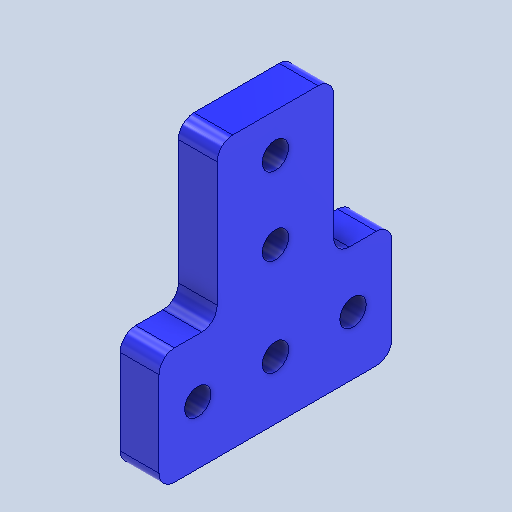
# Autodesk Inventor part: ball_loading_v1_Plate_ASP_F_1
Saved by Autodesk Inventor 2025.1 (Build 291241000, 241)
## iProperties
Created: 2024-11-12
Part Number: ball_loading_v1_Plate_ASP_F_1
Material: ABS プラスチック
Document SubType Name: Modeling
Designer: haruy
Density: 1.06 g/cm^3
Appearance: 青 - 壁塗料 - 光沢
Author: haruy
Autodesk Inventor part; units mm, degrees
ref_plane "YZ Plane" through (0, 0, 0) normal (1, 0, 0) x (0, 1, 0)
ref_plane "XZ Plane" through (0, 0, 0) normal (0, 1, 0) x (-1, 0, 0)
ref_plane "XY Plane" through (0, 0, 0) normal (0, 0, 1) x (1, 0, 0)
sketch "スケッチ1" plane through (0, 0, 0) normal (1, 0, 0) x (0, 1, 0)
  line L0 (-167.5617, 195.4399) -> (192.4383, 195.4399)
  line L1 (192.4383, 195.4399) -> (192.4383, 180.4399)
  line L2 (192.4383, 180.4399) -> (-167.5617, 180.4399)
  line L3 (-167.5617, 180.4399) -> (-167.5617, 195.4399)
  line L4 (-167.5617, 230.4399) -> (-182.5617, 230.4399)
  line L5 (-182.5617, 230.4399) -> (-182.5617, 2.9399)
  line L6 (-182.5617, 2.9399) -> (-167.5617, 2.9399)
  line L7 (-167.5617, 2.9399) -> (-167.5617, 230.4399)
  line L8 (-167.5617, 230.4399) -> (-182.5617, 230.4399)
  line L9 (-182.5617, 230.4399) -> (-182.5617, 215.4399)
  line L10 (-182.5617, 215.4399) -> (-167.5617, 215.4399)
  line L11 (-167.5617, 215.4399) -> (-167.5617, 230.4399)
  line L12 (-117.5617, 180.4399) -> (-102.5617, 180.4399)
  line L13 (-102.5617, 180.4399) -> (-102.5617, 2.9399)
  line L14 (-102.5617, 2.9399) -> (-117.5617, 2.9399)
  line L15 (-117.5617, 2.9399) -> (-117.5617, 180.4399)
  line L16 (192.4383, 180.4399) -> (177.4383, 180.4399)
  line L17 (177.4383, 180.4399) -> (177.4383, 2.9399)
  line L18 (177.4383, 2.9399) -> (192.4383, 2.9399)
  line L19 (192.4383, 2.9399) -> (192.4383, 180.4399)
  circle A0 centre (-142.5617, 135.4399) radius 12.5
  circle A1 centre (-142.5617, 95.4399) radius 18.75
  line L20 (192.4383, 2.9399) -> (-167.5617, 2.9399)
  line L21 (-182.5617, 155.4399) -> (-102.5617, 155.4399)
  line L22 (-102.5617, 75.4399) -> (-182.5617, 75.4399)
  circle A2 centre (-142.5617, 95.4399) radius 20
  line L23 (-125.0617, 195.4399) -> (-125.0617, 180.4399)
  line L24 (-102.5617, 180.4399) -> (-102.5617, 195.4399)
  line L25 (-147.5617, 195.4399) -> (-147.5617, 180.4399)
  line L26 (-167.5617, 202.9399) -> (-182.5617, 202.9399)
  line L27 (-167.5617, 172.9399) -> (-182.5617, 172.9399)
  circle A3 centre (157.4383, 135.4399) radius 12.5
  line L28 (192.4383, 160.4399) -> (177.4383, 160.4399)
  line L29 (169.9383, 195.4399) -> (169.9383, 180.4399)
  line L30 (-167.5617, -189.5601) -> (192.4383, -189.5601)
  line L31 (192.4383, -189.5601) -> (192.4383, -174.5601)
  line L32 (192.4383, -174.5601) -> (-167.5617, -174.5601)
  line L33 (-167.5617, -174.5601) -> (-167.5617, -189.5601)
  line L34 (-167.5617, -224.5601) -> (-182.5617, -224.5601)
  line L35 (-182.5617, -224.5601) -> (-182.5617, 2.9399)
  line L36 (-167.5617, 2.9399) -> (-167.5617, -224.5601)
  line L37 (-167.5617, -224.5601) -> (-182.5617, -224.5601)
  line L38 (-182.5617, -224.5601) -> (-182.5617, -209.5601)
  line L39 (-182.5617, -209.5601) -> (-167.5617, -209.5601)
  line L40 (-167.5617, -209.5601) -> (-167.5617, -224.5601)
  line L41 (-117.5617, -174.5601) -> (-102.5617, -174.5601)
  line L42 (-102.5617, -174.5601) -> (-102.5617, 2.9399)
  line L43 (-117.5617, 2.9399) -> (-117.5617, -174.5601)
  line L44 (192.4383, -174.5601) -> (177.4383, -174.5601)
  line L45 (177.4383, -174.5601) -> (177.4383, 2.9399)
  line L46 (192.4383, 2.9399) -> (192.4383, -174.5601)
  circle A4 centre (-142.5617, -129.5601) radius 12.5
  circle A5 centre (-142.5617, -89.5601) radius 18.75
  line L47 (-182.5617, -149.5601) -> (-102.5617, -149.5601)
  line L48 (-102.5617, -69.5601) -> (-182.5617, -69.5601)
  circle A6 centre (-142.5617, -89.5601) radius 20
  line L49 (-125.0617, -189.5601) -> (-125.0617, -174.5601)
  line L50 (-102.5617, -174.5601) -> (-102.5617, -189.5601)
  line L51 (-147.5617, -189.5601) -> (-147.5617, -174.5601)
  line L52 (-167.5617, -197.0601) -> (-182.5617, -197.0601)
  line L53 (-167.5617, -167.0601) -> (-182.5617, -167.0601)
  circle A7 centre (157.4383, -129.5601) radius 12.5
  line L54 (192.4383, -154.5601) -> (177.4383, -154.5601)
  line L55 (169.9383, -189.5601) -> (169.9383, -174.5601)
  line L56 (192.4383, 155.4399) -> (144.9383, 155.4399)
  line L57 (144.9383, 155.4399) -> (144.9383, 75.4399)
  line L58 (144.9383, 75.4399) -> (192.4383, 75.4399)
  line L59 (192.4383, 75.4399) -> (192.4383, 155.4399)
  line L60 (177.4383, 155.4399) -> (153.4158, 147.275)
  line L61 (146.595, 129.2213) -> (177.4383, 75.4399)
  circle A8 centre (-175.0617, 197.9399) radius 1.7
  circle A9 centre (-175.0617, 187.9399) radius 1.7
  circle A10 centre (-175.0617, 177.9399) radius 1.7
  circle A11 centre (-162.5617, 187.9399) radius 1.7
  circle A12 centre (-152.5617, 187.9399) radius 1.7
  point P0 (0, 0)
  point P1 (-120.0617, 187.9399)
  point P2 (-110.0617, 187.9399)
  point P3 (-110.0617, 175.4399)
  point P4 (-110.0617, 165.4399)
  point P5 (184.9383, 175.4399)
  point P6 (184.9383, 165.4399)
  point P7 (184.9383, 187.9399)
  point P8 (174.9383, 187.9399)
  point P9 (-110.0617, 180.4399)
  point P10 (192.4383, 187.9399)
  point P11 (-110.0617, 95.4399)
  point P12 (-110.0617, 135.4399)
  point P13 (-175.0617, 135.4399)
  point P14 (-175.0617, 95.4399)
  point P15 (-175.0617, -89.5601)
  point P16 (-110.0617, -89.5601)
  point P17 (-110.0617, -129.5601)
  point P18 (-175.0617, -129.5601)
  point P19 (-175.0617, -172.0601)
  point P20 (-175.0617, -182.0601)
  point P21 (-175.0617, -192.0601)
  point P22 (-162.5617, -182.0601)
  point P23 (-152.5617, -182.0601)
  point P24 (-120.0617, -182.0601)
  point P25 (-110.0617, -182.0601)
  point P26 (-110.0617, -169.5601)
  point P27 (-110.0617, -159.5601)
  point P28 (174.9383, -182.0601)
  point P29 (184.9383, -182.0601)
  point P30 (184.9383, -169.5601)
  point P31 (184.9383, -159.5601)
  point P32 (184.9383, 135.4399)
  point P33 (184.9383, 95.4399)
  point P34 (177.4383, 91.6899)
  point P35 (184.9383, -89.5601)
  point P36 (184.9383, -129.5601)
  dimension "d0" = 7.5
  dimension "d1" = 7.5
  dimension "d2" = 7.5
  dimension "d3" = 7.5
  dimension "d4" = 10
  dimension "d5" = 10
  dimension "d6" = 5
  dimension "d7" = 10
  dimension "d8" = 7.5
  dimension "d9" = 7.5
  dimension "d10" = 7.5
  dimension "d11" = 10
  dimension "d12" = 7.5
  dimension "d13" = 7.5
  dimension "d14" = 5
  dimension "d15" = 10
  dimension "d16" = 7.5
  dimension "d17" = 7.5
  dimension "d18" = 7.5
  dimension "d19" = 10
  dimension "d20" = 7.5
  dimension "d21" = 7.5
  dimension "d22" = 5
  dimension "d23" = 10
  dimension "d24" = 7.5
  dimension "d25" = 7.5
  dimension "d26" = 20
  dimension "d27" = 20
  dimension "d28" = 7.5
  dimension "d29" = 7.5
  dimension "d30" = 20
  dimension "d31" = 7.5
  dimension "d32" = 7.5
  dimension "d33" = 20
  dimension "d34" = 3.4
  dimension "d35" = 3.4
  dimension "d36" = 3.4
  dimension "d37" = 3.4
  dimension "d38" = 3.4
  constraints: 124 end point, 19 symmetric about line, 13 centre point, 5 coincident, 2 midpoint
  measures "d0" distance from line of L3 point (-175.062, 187.94)
  measures "d1" distance from line of point (-175.062, 197.94) L7
  measures "d2" distance from line of L7 point (-175.062, 177.94)
  measures "d3" distance from line of L2 point (-175.062, 187.94)
  measures "d4" distance of point (-175.062, 197.94) point (-175.062, 187.94)
  measures "d5" distance of point (-175.062, 177.94) point (-175.062, 187.94)
  measures "d6" distance from line of point (-162.562, 187.94) L3
  measures "d7" distance of point (-152.562, 187.94) point (-162.562, 187.94)
  measures "d8" distance from line of point (-162.562, 187.94) L0
  measures "d9" distance from line of L2 point (-152.562, 187.94)
  measures "d10" distance from line of point (-120.062, 187.94) L0
  measures "d11" distance of point (-110.062, 187.94) point (-120.062, 187.94)
  measures "d12" distance from line of L24 point (-110.062, 187.94)
  measures "d13" distance from line of L12 point (-110.062, 187.94)
  measures "d14" distance of point (-110.062, 175.44) point (-110.062, 180.44)
  measures "d15" distance of point (-110.062, 165.44) point (-110.062, 175.44)
  measures "d16" distance from line of point (-110.062, 175.44) L15
  measures "d17" distance from line of point (-110.062, 165.44) L15
  measures "d18" distance of point (192.438, 187.94) point (184.938, 187.94)
  measures "d19" distance of point (174.938, 187.94) point (184.938, 187.94)
  measures "d20" distance from line of point (174.938, 187.94) L0
  measures "d21" distance from line of L0 point (184.938, 187.94)
  measures "d22" distance from line of point (184.938, 175.44) L16
  measures "d23" distance of point (184.938, 165.44) point (184.938, 175.44)
  measures "d24" distance from line of L19 point (184.938, 175.44)
  measures "d25" distance from line of L19 point (184.938, 165.44)
  measures "d26" distance from line of L21 point (-110.062, 135.44)
  measures "d27" distance from line of L22 point (-110.062, 95.44)
  measures "d28" distance from line of L15 point (-110.062, 95.44)
  measures "d29" distance from line of L15 point (-110.062, 135.44)
  measures "d30" distance from line of L21 point (-175.062, 135.44)
  measures "d31" distance from line of point (-175.062, 135.44) L5
  measures "d32" distance from line of point (-175.062, 95.44) L5
  measures "d33" distance from line of L22 point (-175.062, 95.44)
  measures "d34" diameter of A8
  measures "d35" diameter of A9
  measures "d36" diameter of A10
  measures "d37" diameter of A11
  measures "d38" diameter of A12
extrude "押し出し1" add sketch "スケッチ1" along normal blind 5 contours L0 L25 L2 L3 | L3 L7 L27 L5 L26
fillet "フィレット1" radius 2 8 edges at (2.5, -147.5617, 195.4399) (2.5, -167.5617, 195.4399) (2.5, -167.5617, 202.9399) (2.5, -182.5617, 202.9399) (2.5, -182.5617, 172.9399) (2.5, -167.5617, 172.9399) (2.5, -167.5617, 180.4399) (2.5, -147.5617, 180.4399)
equation "\"d1\" = d0"
equation "\"d2\" = d0"
equation "\"d3\" = d0"
equation "\"d8\" = d0"
equation "\"d9\" = d0"
equation "\"d10\" = d0"
equation "\"d12\" = d0"
equation "\"d13\" = d0"
equation "\"d16\" = d0"
equation "\"d17\" = d0"
equation "\"d20\" = d18"
equation "\"d21\" = d18"
equation "\"d24\" = d18"
equation "\"d25\" = d18"
equation "\"d32\" = d31"
equation "\"d33\" = d30"
